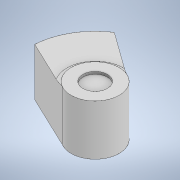
# Autodesk Inventor part: elementy_dodatkowe
Saved by Autodesk Inventor 2020 (Build 240168000, 168)
## iProperties
Created: 2019-12-28
Part Number: elementy_dodatkowe
Material: Ogólny
Document SubType Name: Modeling
Designer: macie
Density: 1 g/cm^3
Appearance: Domyślna
Author: macie
## iProperties of the stored document _Drukowanie 3D.ipt
Created: 2019-12-29
Part Number: _Drukowanie 3D
Material: Ogólny
Document SubType Name: Modeling
Designer: macie
Density: 1 g/cm^3
Appearance: Domyślna
Author: macie
Autodesk Inventor part; units mm, degrees
ref_plane "YZ Plane" through (0, 0, 0) normal (1, 0, 0) x (0, 1, 0)
ref_plane "XZ Plane" through (0, 0, 0) normal (0, 1, 0) x (-1, 0, 0)
ref_plane "XY Plane" through (0, 0, 0) normal (0, 0, 1) x (1, 0, 0)
sketch "Szkic1" plane through (0, 0, 0) normal (0, 1, 0) x (-1, 0, 0)
  line L0 (-125.2393, -14.1807) -> (-26.2247, 164.0455)
  arc A0 (-125.2393, -14.1807) -> (-99.0146, -58.75) centre (-99.0146, -28.75) ccw
  line L1 (99.0146, -58.75) -> (-99.0146, -58.75)
  line L2 (26.2247, 164.0455) -> (125.2393, -14.1807)
  arc A1 (26.2247, 164.0455) -> (-26.2247, 164.0455) centre (0, 149.4762) ccw
  line L3 (-23.6022, 162.5886) -> (-122.6168, -15.6376)
  arc A2 (-122.6168, -15.6376) -> (-99.0146, -55.75) centre (-99.0146, -28.75) ccw
  line L4 (-99.0146, -55.75) -> (99.0146, -55.75)
  arc A3 (113.6938, -51.4109) -> (125.9544, -30.5508) centre (99.0146, -28.75) ccw
  line L5 (122.6168, -15.6376) -> (23.6022, 162.5886)
  arc A4 (23.6022, 162.5886) -> (-23.6022, 162.5886) centre (0, 149.4762) ccw
  circle A5 centre (99.0146, -28.75) radius 5.1
  arc A6 (104.1146, -20.1483) -> (94.9151, -37.8711) centre (99.0146, -28.75) ccw
  line L6 (104.1146, -20.1483) -> (125.9544, -30.5508)
  line L7 (94.9151, -37.8711) -> (113.6938, -51.4109)
  arc A7 (99.0146, -58.75) -> (116.2857, -53.2797) centre (99.0146, -28.75) ccw
  arc A8 (128.8458, -31.9279) -> (125.2393, -14.1807) centre (99.0146, -28.75) ccw
  point P0 (0, 0)
  point P1 (0, 0)
  dimension "d0" = 3
  dimension "d1" = 10.2
  dimension "d2" = 20
  constraints: 16 end point, 16 point on circle, 9 centre point, 2 point on line, 1 coincident, 3 other
  measures "d0" distance between parallel lines of L0 L3
  measures "d1" diameter of A5
  measures "d2" diameter of A6
extrude "Wyciągnięcie proste1" add sketch "Szkic1" along normal blind 5
sketch "Szkic2" plane through (0, 5, 0) normal (0, 1, 0) x (1, 0, 0)
  circle A0 centre (-99.0146, 28.75) radius 5.1 projected
  circle A1 centre (-99.0146, 28.75) radius 5.1
  point P0 (0, 0)
  constraints: 1 centre point, 1 coincident
extrude "Wyciągnięcie proste2" add sketch "Szkic2" against normal blind 5
sketch "Szkic3" plane through (0, 5, 0) normal (0, 1, 0) x (1, 0, 0)
  arc A0 (-104.1146, 20.1483) -> (-94.9151, 37.8711) centre (-99.0146, 28.75) ccw projected
  circle A1 centre (-99.0146, 28.75) radius 5.1
  circle A2 centre (-99.0146, 28.75) radius 10
  point P0 (0, 0)
  point P1 (-94.9151, 37.8711)
  dimension "d7" = 10.2
  constraints: 2 centre point, 2 coincident
  measures "d7" diameter of A1
extrude "Wyciągnięcie proste3" add sketch "Szkic3" along normal blind 1
fillet "Zaokrąglenie1" radius 2 1 edges at (-107.8901, 5, -33.357)
sketch "Szkic4" plane through (0, 0, 0) normal (0, -1, 0) x (1, 0, 0)
  line L0 (-94.9151, -37.8711) -> (-113.6938, -51.4109) projected
  arc A0 (-94.9151, -37.8711) -> (-104.1146, -20.1483) centre (-99.0146, -28.75) ccw projected
  line L1 (-125.9544, -30.5508) -> (-104.1146, -20.1483) projected
  arc A1 (-125.9544, -30.5508) -> (-113.6938, -51.4109) centre (-99.0146, -28.75) ccw projected
  point P0 (0, 0)
extrude "Wyciągnięcie proste4" add sketch "Szkic4" along normal blind 15
